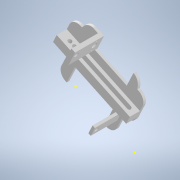
# Autodesk Inventor part: s_support_bottom
Saved by Autodesk Inventor 2020.1 (Build 241239000, 239)
## iProperties
Created: 2019-10-17
Part Number: s_support_bottom
Material: Generic
Document SubType Name: Modeling
Designer: jesse
Density: 1 g/cm^3
Appearance: Default
support_length: 2.300 in
hole_size: 0.118 in
Author: jesse
## iProperties of the stored document _3DPrint.ipt
Created: 2019-10-25
Part Number: _3DPrint
Material: Generic
Document SubType Name: Modeling
Designer: jesse
Density: 1 g/cm^3
Appearance: Default
Author: jesse
Autodesk Inventor part; units mm, degrees
ref_plane "YZ Plane" through (0, 0, 0) normal (1, 0, 0) x (0, 1, 0)
ref_plane "XZ Plane" through (0, 0, 0) normal (0, 1, 0) x (-1, 0, 0)
ref_plane "XY Plane" through (0, 0, 0) normal (0, 0, 1) x (1, 0, 0)
ref_plane "Work Plane1" through (19.722, 36.341, 0) normal (0, 0, 1) x (0.4250843, 0.9051538, 0)
sketch "Sketch1" plane through (19.722, 36.341, 0) normal (0, 0, 1) x (0.4250843, 0.9051538, 0)
  line L0 (-12.1227, 70.1452) -> (-18.8796, 70.1452)
  line L1 (-18.8796, 70.1452) -> (-18.8796, 11.7252)
  line L2 (-18.8796, 11.7252) -> (-12.1227, 11.7252)
  line L3 (-12.1227, 11.7252) -> (-12.1227, 70.1452)
  point P0 (-41.2777, 2.4034)
  dimension "support_length" = 58.42
  constraints: 8 end point, 2 parallel, 1 horizontal, 1 perpendicular
  measures "support_length" distance of L2.end L0.start
extrude "Extrusion1" add sketch "Sketch1" along normal blind 8
sketch "Sketch2" plane through (1.0834, 24.2363, 0) normal (-0.4250843, -0.9051538, 0) x (0, 0, 1)
  line L0 (0, 58.42) -> (8, 58.42) construction
  line L1 (4, 58.42) -> (4, 0) construction
  line L2 (0, 0) -> (8, 0) construction
  line L3 (4, 52.42) -> (4, 5) construction
  line L4 (2.5, 52.42) -> (2.5, 5)
  line L5 (5.5, 5) -> (5.5, 52.42)
  arc A0 (5.5, 52.42) -> (2.5, 52.42) centre (4, 52.42) ccw
  arc A1 (2.5, 5) -> (5.5, 5) centre (4, 5) ccw
  line L6 (4, 5) -> (6.3728, 5) construction
  line L7 (4, 52.42) -> (6.6371, 52.42) construction
  line L8 (5.634, 5) -> (5.634, 0) construction
  circle A2 centre (4, 56.42) radius 1.5
  line L9 (4, 56.42) -> (7.1435, 56.42) construction
  point P0 (0, -9.3218)
  point P1 (4, 28.71)
  dimension "d5" = 3
  dimension "d6" = 3
  dimension "d7" = 2
  dimension "d8" = 5
  dimension "d9" = 4
  constraints: 18 end point, 5 point on line, 4 point on circle, 4 tangent, 3 centre point, 3 horizontal, 3 midpoint, 1 parallel
  measures "d5" distance between parallel lines of L4 L5
  measures "d6" diameter of A2
  measures "d7" distance between parallel lines of L9 L0
  measures "d8" distance between parallel lines of L6 L2
  measures "d9" distance between parallel lines of L7 L9
extrude "Extrusion2" cut sketch "Sketch2" against normal blind 15.875
sketch "Sketch3" plane through (19.722, 36.341, 0) normal (0, 0, -1) x (-0.9051538, 0.4250843, 0)
  line L0 (70.1452, -12.1227) -> (70.1452, -18.8796) construction
  line L1 (11.7252, -12.1227) -> (70.1452, -12.1227) construction
  line L2 (70.1452, -18.8796) -> (11.7252, -12.1227) construction
  line L3 (70.1452, -4.7378) -> (11.7252, -4.7378)
  line L4 (11.7252, -4.7378) -> (11.7252, -26.2645)
  line L5 (11.7252, -26.2645) -> (70.1452, -26.2645)
  line L6 (70.1452, -26.2645) -> (70.1452, -4.7378)
  line L7 (70.1452, -4.7378) -> (11.7252, -26.2645) construction
  line L8 (11.7252, -4.7378) -> (70.1452, -26.2645) construction
  line L9 (11.7252, -18.8796) -> (11.7252, -12.1227) projected
  point P0 (2.4034, -41.2777)
  point P1 (40.9352, -15.5011)
  constraints: 14 end point, 3 midpoint, 2 parallel, 1 collinear, 1 horizontal, 1 perpendicular
extrude "Extrusion3" add sketch "Sketch3" along normal blind 2
ref_plane "Work Plane7" through (-28.3656, 60.8921, 2.8116) normal (-0.9051538, 0.4250843, 0) x (-0.4250843, -0.9051538, 0)
sketch "Sketch12" plane through (-28.3656, 60.8921, 2.8116) normal (-0.9051538, 0.4250843, 0) x (-0.4250843, -0.9051538, 0)
  line L0 (28.0457, -4.8116) -> (6.519, -4.8116) projected
  line L1 (-6.0189, 5.1884) -> (7.4039, 5.1884)
  line L2 (7.4039, 5.1884) -> (7.4039, -4.8116)
  line L3 (7.4039, -4.8116) -> (-6.0189, -4.8116)
  line L4 (-6.0189, -4.8116) -> (-6.0189, 5.1884)
  line L5 (13.9039, 5.1884) -> (20.6608, 5.1884) projected
  line L6 (13.9039, -2.8116) -> (13.9039, 5.1884) projected
  point P0 (43.0589, -2.8116)
  point P1 (7.4039, -4.8116)
  dimension "d30" = 6.5
  dimension "d31" = 13.4228
  constraints: 8 end point, 2 collinear, 2 parallel, 1 horizontal, 1 perpendicular
  measures "d30" distance between parallel lines of L2 L6
  measures "d31" distance of L1.start L1.end
extrude "Extrusion11" add sketch "Sketch12" along normal blind 3.175
sketch "Sketch13" plane through (19.722, 36.341, -2) normal (0, 0, -1) x (-0.9051538, 0.4250843, 0)
  line L0 (2.4034, 29.2184) -> (85.4586, 29.2184)
  line L1 (85.4586, 29.2184) -> (85.4586, -51.6034)
  line L2 (85.4586, -51.6034) -> (2.4034, -51.6034)
  line L3 (2.4034, -51.6034) -> (2.4034, 29.2184)
  point P0 (2.4034, -51.6034)
  constraints: 8 end point, 2 parallel, 1 coincident, 1 horizontal, 1 perpendicular
extrude "Bottom Add" add sketch "Sketch13" against normal up to surface (2 mm away)
sketch "Sketch14" plane through (19.722, 36.341, -2) normal (0, 0, -1) x (-0.9051538, 0.4250843, 0)
  line L0 (26.4629, 4.0975) -> (26.4629, -2.5351) projected
  line L1 (53.9629, -5.6227) -> (53.9629, 7.8001) projected
  line L2 (53.9629, -5.6227) -> (57.1379, -5.6227) projected
  line L3 (53.9629, 7.8001) -> (26.2629, 7.8001)
  line L4 (26.2629, 7.8001) -> (26.2629, -5.6227)
  line L5 (26.2629, -5.6227) -> (53.9629, -5.6227)
  line L6 (53.9629, -5.6227) -> (53.9629, 7.8001)
  point P0 (2.4034, -41.2777)
  point P1 (53.9629, -5.6227)
  dimension "d72" = 0.2
  constraints: 8 end point, 2 parallel, 1 horizontal, 1 perpendicular
  measures "d72" distance between parallel lines of L4 L0
extrude "Extrusion13" cut sketch "Sketch14" against normal blind 11.1125
sketch "Sketch15" plane through (-31.2395, 62.2417, 2.8116) normal (-0.9051538, 0.4250843, 0) x (0, 0, 1)
  circle A0 centre (0.1884, 3.5) radius 0.625 projected
  circle A1 centre (0.1884, -5.5) radius 0.625 projected
  circle A2 centre (0.1884, -1) radius 2 projected
  point P0 (-2.8116, -43.0589)
extrude "Extrusion14" cut sketch "Sketch15" against normal blind 25.4
ref_plane "Midplane of Slot" through (-3.4424, 26.3617, 4) normal (0, 0, -1) x (-0.9051538, 0.4250843, 0)
move faces "Move1" translate (0, 0, 12.86) faces at (-29.6249, 63.19, 8) (-32.4708, 54.6403, 2.6667)
sketch "Sketch17" plane through (19.722, 36.341, 0) normal (0, 0, 1) x (0.9051538, -0.4250843, 0)
  point P0 (-2.4034, -41.2777)
ref_plane "Work Plane9" through (-41.6263, 85.4913, -2) normal (0, 0, 1) x (-0.9051538, 0.4250843, 0)
sketch "Sketch19" plane through (19.722, 36.341, 0) normal (0, 0, 1) x (0.9051538, -0.4250843, 0)
  line L0 (-19.4861, -0.6396) -> (-18.3292, -0.6396) projected
  ellipse E0 centre (-25.9492, -2.5583) end of major axis (-25.9492, 6.7812) minor radius 6.604 (-19.4861, -0.6396) -> (-25.9492, 6.7812) ccw projected
  line L1 (-25.9492, 6.7812) -> (-61.0012, 6.7812) projected
  ellipse E1 centre (-61.0012, -2.5583) end of major axis (-61.0012, -11.8977) minor radius 6.604 (-61.0012, 6.7812) -> (-67.4644, -0.6396) ccw projected
  line L2 (-68.6212, -0.6396) -> (-67.4644, -0.6396) projected
  arc A0 (-68.6212, -0.6396) -> (-75.2252, -7.2436) centre (-68.6212, -7.2436) ccw projected
  line L3 (-75.2252, -7.2436) -> (-75.2252, -19.4356) projected
  arc A1 (-75.2252, -19.4356) -> (-68.6212, -26.0396) centre (-68.6212, -19.4356) ccw projected
  line L4 (-67.6052, -26.0396) -> (-68.6212, -26.0396) projected
  line L5 (-67.6052, -38.4856) -> (-67.6052, -26.0396) projected
  arc A2 (-67.6052, -38.4856) -> (-61.0012, -45.0896) centre (-61.0012, -38.4856) ccw projected
  line L6 (-61.0012, -45.0896) -> (-25.9492, -45.0896) projected
  arc A3 (-25.9492, -45.0896) -> (-19.3452, -38.4856) centre (-25.9492, -38.4856) ccw projected
  line L7 (-19.3452, -26.0396) -> (-19.3452, -38.4856) projected
  line L8 (-18.3292, -26.0396) -> (-19.3452, -26.0396) projected
  arc A4 (-18.3292, -26.0396) -> (-11.7252, -19.4356) centre (-18.3292, -19.4356) ccw projected
  line L9 (-11.7252, -7.2436) -> (-11.7252, -19.4356) projected
  arc A5 (-11.7252, -7.2436) -> (-18.3292, -0.6396) centre (-18.3292, -7.2436) ccw projected
  line L10 (-121.61, -93.4487) -> (41.8687, -93.4487)
  line L11 (41.8687, -93.4487) -> (41.8687, 56.8332)
  line L12 (41.8687, 56.8332) -> (-121.61, 56.8332)
  line L13 (-121.61, 56.8332) -> (-121.61, -93.4487)
  point P0 (-2.4034, -41.2777)
  constraints: 8 end point, 2 parallel, 1 horizontal, 1 perpendicular, 2 other
extrude "Bottom Cutout" cut sketch "Sketch19" against normal mid plane 42.8625
sketch "Sketch20" plane through (19.722, 36.341, 0) normal (0, 0, 1) x (0.9051538, -0.4250843, 0)
  line L0 (-11.7252, -26.0396) -> (-26.3452, -26.0396) construction
  line L1 (-23.3452, -26.0396) -> (-21.3452, -26.0396)
  line L2 (-21.3452, -26.0396) -> (-21.3452, -33.6596)
  line L3 (-21.3452, -33.6596) -> (-23.3452, -33.6596)
  line L4 (-23.3452, -33.6596) -> (-23.3452, -26.0396)
  line L5 (-19.3452, -33.6596) -> (-20.9464, -33.6596) construction
  line L6 (-19.3452, -38.4856) -> (-19.3452, -26.0396) construction
  point P0 (-2.4034, -41.2777)
  dimension "d48" = 2
  dimension "d49" = 2
  constraints: 10 end point, 2 horizontal, 2 parallel, 1 collinear, 1 perpendicular, 1 point on line, 1 other
  measures "d48" distance between parallel lines of L6 L2
  measures "d49" distance of L2.end L3.end
ref_plane "Work Plane10" through (-12.098, 10.8554, 20.86) normal (0, 0, 1) x (0.9051538, -0.4250843, 0)
extrude "Extrusion16" add sketch "Sketch20" along normal up to surface (20.86 mm away)
sketch "Sketch22" plane through (19.722, 36.341, 0) normal (0, 0, 1) x (0.9051538, -0.4250843, 0)
  line L0 (-59.6042, -55.8846) -> (-59.6042, -37.8506) construction
  line L1 (-27.3462, -37.8506) -> (-27.3462, -55.8846) construction
  line L2 (-36.6172, -30.1544) -> (-50.3332, -30.1544) construction
  line L3 (-59.9042, -29.8544) -> (-27.0462, -29.8544)
  line L4 (-27.0462, -29.8544) -> (-27.0462, -57.6532)
  line L5 (-27.0462, -57.6532) -> (-59.9042, -57.6532)
  line L6 (-59.9042, -57.6532) -> (-59.9042, -29.8544)
  point P0 (-2.4034, -41.2777)
  dimension "d54" = 0.3
  dimension "d55" = 0.3
  dimension "d56" = 0.3
  dimension "d57" = 27.7988
  constraints: 8 end point, 2 parallel, 1 horizontal, 1 perpendicular
  measures "d54" distance between parallel lines of L0 L6
  measures "d55" distance between parallel lines of L2 L3
  measures "d56" distance between parallel lines of L1 L4
  measures "d57" distance between parallel lines of L3 L5
extrude "Extrusion18" cut sketch "Sketch22" against normal blind 26.9875
sketch "Sketch23" plane through (-12.4781, 22.6949, 0) normal (-0.9051538, 0.4250843, 0) x (0, 0, 1)
  circle A0 centre (17.685, -3.81) radius 1.5875 projected
  point P0 (0, -15.2381)
extrude "Extrusion19" cut sketch "Sketch23" against normal blind 6.35
sketch "Sketch24" plane through (-28.3656, 60.8921, 2.8116) normal (0.9051538, -0.4250843, 0) x (0, 0, -1)
  point P0 (2.8116, -43.0589)
sketch "Sketch25" plane through (-28.3656, 60.8921, 2.8116) normal (0.9051538, -0.4250843, 0) x (0, 0, -1)
  circle A0 centre (-14.8734, 0.3218) radius 1.5875 projected
  point P0 (2.8116, -43.0589)
extrude "Extrusion20" cut sketch "Sketch25" against normal blind 25.4
move faces "Move2" translate (-1.4484, 0.6802, 0) faces at (-49.8808, 53.1471, 2.6667)
move faces "Move3" translate (-3.1498, 1.4792, 0) faces at (-51.3293, 53.8273, 2.6667)
equation "\"d5\" = hole_size"
equation "\"d6\" = hole_size"
equation "\"hole_size\" = 3"
body "Solid1"
